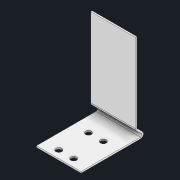
# Autodesk Inventor part: LaminaResorte
Saved by Autodesk Inventor 2021 (Build 250183000, 183)
## iProperties
Created: 2021-06-15
Part Number: LaminaResorte
Material: Stainless Steel
Document SubType Name: Sheet Metal
Designer: GABRIEL LOL
Density: 8 g/cm^3
Sheet Metal Rule: Por defecto_mm
Appearance: White
Flat Pattern Width: 1.5 cm
Flat Pattern Length: 5.14335 cm
Flat Pattern Area: 7.71503 cm^2
Sheet Metal Width: 15.000 mm
Sheet Metal Length: 51.434 mm
Sheet Metal Area: 771.503 mm^2
Author: GABRIEL LOL
Autodesk Inventor part; units mm, degrees
ref_plane "YZ Plane" through (0, 0, 0) normal (1, 0, 0) x (0, 1, 0)
ref_plane "XZ Plane" through (0, 0, 0) normal (0, 1, 0) x (-1, 0, 0)
ref_plane "XY Plane" through (0, 0, 0) normal (0, 0, 1) x (1, 0, 0)
sketch "Sketch1" plane through (0, 0, 0) normal (0, 1, 0) x (-1, 0, 0)
  line L0 (0, 4.9984) -> (-15, 4.9984)
  line L1 (-15, 4.9984) -> (-15, -15.0016)
  line L2 (-15, -15.0016) -> (0, -15.0016)
  line L3 (0, -15.0016) -> (0, 4.9984)
  dimension "d0" = 15
  dimension "d1" = 20
  measures "d0" distance of L2.end L1.end
  measures "d1" distance of L1.end L0.end
extrude "Plate1" add sketch "Sketch1" along normal blind 0.5
sketch "Sketch2" plane through (0, 1.3536, -15.3552) normal (0, 0.7071068, -0.7071068) x (-1, 0, 0)
  line L0 (-15, 0) -> (0, 0)
  line L1 (0, 0) -> (0, 2.5858)
  line L2 (0, 2.5858) -> (-15, 2.5858)
  line L3 (-15, 2.5858) -> (-15, 0)
  constraints: 6 end point, 1 horizontal, 1 perpendicular, 1 vertical
edge flange "Flange1" height 5 angle 135 thickness 0.5 bend radius 0.5 thickness toward (0, 0.7071068, -0.7071068) relief tear relief width 0.5 relief depth 0.25 edges at (7.5, 0.5, -15.0016) wall of the first edge with corners at (15, 1.3536, -15.3552) (0, 1.3536, -15.3552) (0, 3.182, -13.5267) (15, 3.182, -13.5267)
bend "Bend1"
corner "Corner1"
sketch "Sketch3" plane through (15, 3.8891, -13.7338) normal (0, 0, 1) x (1, 0, 0)
  line L0 (-15, 0) -> (0, 0)
  line L1 (0, 0) -> (0, 26.5858)
  line L2 (0, 26.5858) -> (-15, 26.5858)
  line L3 (-15, 26.5858) -> (-15, 0)
  constraints: 6 end point, 1 horizontal, 1 perpendicular, 1 vertical
edge flange "Flange2" height 27 angle 45 thickness 0.5 bend radius 0.5 thickness toward (0, 0, 1) relief tear relief width 0.5 relief depth 0.25 edges at (7.5, 3.5355, -13.8803) wall of the first edge with corners at (0, 3.8891, -13.7338) (15, 3.8891, -13.7338) (15, 30.4749, -13.7338) (0, 30.4749, -13.7338)
bend "Bend2"
corner "Corner2"
sketch "Sketch4" plane through (0, 0, 0) normal (0, -1, 0) x (1, 0, 0)
  circle A0 centre (10, 2.4984) radius 1 projected
  circle A1 centre (5, 2.4984) radius 1 projected
  circle A2 centre (5, -7.5016) radius 1 projected
  circle A3 centre (10, -7.5016) radius 1 projected
  point P0 (0, 0)
extrude "Extrusion1" cut sketch "Sketch4" against normal blind 10
equation "\"d2\" = Thickness"
equation "\"d3\" = BendReliefWidth"
equation "\"d4\" = BendReliefDepth"
equation "\"d5\" = MinimumRemnant"
equation "\"d6\" = TransitionRadius"
equation "\"d9\" = BendRadius"
equation "\"d10\" = CornerReliefSize"
equation "\"d11\" = GapSize"
equation "\"d12\" = JacobiRadiusSize"
equation "\"d13\" = BendReliefWidth"
equation "\"d14\" = BendReliefDepth"
equation "\"d15\" = MinimumRemnant"
equation "\"d16\" = TransitionRadius"
equation "\"d19\" = BendRadius"
equation "\"d20\" = CornerReliefSize"
equation "\"d21\" = GapSize"
equation "\"d22\" = JacobiRadiusSize"
equation "\"BendRadius\" = Thickness"
equation "\"BendReliefWidth\" = Thickness"
equation "\"BendReliefDepth\" = 0.5 * Thickness"
equation "\"CornerReliefSize\" = 4 * Thickness"
equation "\"MinimumRemnant\" = 2 * Thickness"
equation "\"TransitionRadius\" = BendRadius"
equation "\"JacobiRadiusSize\" = BendRadius"
equation "\"GapSize\" = Thickness"
equation "\"Thickness\" = 0.5"
body "Solid1"
